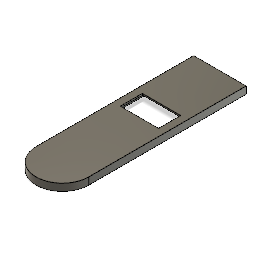
M365_panel_windowed (Autodesk Fusion 360 design; units mm, degrees)
Autodesk Fusion 360 part; units mm, degrees
sketch "Sketch1" plane through (0, 0, 0) normal (0, 1, 0) x (1, 0, 0)
  line L0 (-16.3, 0) -> (16.3, 0)
  line L1 (16.3, 0) -> (16.3, 97.5)
  line L2 (16.3, 97.5) -> (-16.3, 97.5)
  line L3 (-16.3, 97.5) -> (-16.3, 0)
  line L4 (0, 102.6744) -> (0, -20) construction
  arc A0 (-16.3, 0) -> (16.3, 0) centre (0, 0) ccw
  line L5 (-14.35, 97.5) -> (-14.35, 0)
  arc A1 (-14.35, 0) -> (14.35, 0) centre (0, 0) ccw
  line L6 (14.35, 0) -> (14.35, 97.5)
  dimension "d1" = 32.6
  dimension "d2" = 97.5
  dimension "d3" = 1.95
  measures "d3" distance of L3
extrude "Extrude1" add sketch "Sketch1" along normal blind 2
extrude "Extrude2" add sketch "Sketch1" against normal blind 2.5 contours L0 L2 L3 L5 | L0 A0 A1 | L0 L1 L2 L6
sketch "Sketch2" plane through (0, 0, 7.15) normal (0, 1, 0) x (1, 0, 0)
  circle A0 centre (0, 7.15) radius 3.5
  circle A1 centre (0, 7.15) radius 4.1
  circle A2 centre (0, 7.15) radius 4.7
  circle A3 centre (0, 7.15) radius 5.3
  circle A4 centre (0, 7.15) radius 5.9
  circle A5 centre (0, 7.15) radius 6.5
  circle A6 centre (0, 7.15) radius 7.1
  circle A7 centre (0, 7.15) radius 7.7
  circle A8 centre (0, 7.15) radius 8.3
  line L0 (27.1083, -9.4638) -> (28.3083, -9.4638)
  line L1 (28.3083, -9.4638) -> (28.3083, -7.488)
  line L2 (28.3083, -7.488) -> (27.1083, -7.488)
  line L3 (27.1083, -7.488) -> (27.1083, -9.4638)
  circle A9 centre (0, 7.15) radius 8.9
  circle A10 centre (0, 7.15) radius 9.5
  circle A11 centre (0, 7.15) radius 10.1
  circle A12 centre (0, 7.15) radius 10.7
  circle A13 centre (0, 7.15) radius 11.3
  circle A14 centre (0, 7.15) radius 11.9
  circle A15 centre (0, 7.15) radius 12.5
  dimension "d18" = 7
  dimension "d19" = 8.2
  dimension "d20" = 1.2
  dimension "d21" = 9.4
  dimension "d22" = 10.6
  dimension "d23" = 11.8
  dimension "d24" = 13
  dimension "d25" = 14.2
  dimension "d26" = 15.4
  dimension "d27" = 16.6
  dimension "d28" = 17.8
  dimension "d29" = 19
  dimension "d30" = 20.2
  dimension "d31" = 21.4
  dimension "d32" = 22.6
  dimension "d33" = 23.8
  dimension "d34" = 25
  measures "d18" diameter of A0
  measures "d19" diameter of A1
  measures "d21" diameter of A2
  measures "d22" diameter of A3
  measures "d23" diameter of A4
  measures "d24" diameter of A5
  measures "d25" diameter of A6
  measures "d26" diameter of A7
  measures "d27" diameter of A8
  measures "d28" diameter of A9
  measures "d29" diameter of A10
  measures "d30" diameter of A11
  measures "d31" diameter of A12
  measures "d32" diameter of A13
  measures "d33" diameter of A14
  measures "d34" diameter of A15
extrude "Extrude4" cut sketch "Sketch2" along normal blind 1.25 contours A1 | A2 | A3 | A4 | A5 | A6 | A7 | A8 | A9 | A10 | A11 | A12 | A13 | A14 | A15
extrude "Extrude5" add 1 faces at (0.555, 0, 0.9381) along direction (0, -1, 0) blind 1.5
sketch "Sketch3" plane through (0, 0, 0) normal (0, -1, 0) x (1, 0, 0)
  line L0 (14.35, -97.5) -> (14.35, 0)
  arc A0 (14.35, 0) -> (-14.35, 0) centre (0, 0) ccw
  line L1 (-14.35, 0) -> (-14.35, -97.5)
  line L2 (-14.35, -97.5) -> (14.35, -97.5)
  circle A1 centre (0, 0) radius 12.5
  line L3 (13, -62.5) -> (-13, -62.5)
  line L4 (-13, -62.5) -> (-13, -46.5)
  line L5 (-13, -46.5) -> (13, -46.5)
  line L6 (13, -46.5) -> (13, -62.5)
  line L7 (13, -62.5) -> (-13, -46.5) construction
  line L8 (-13, -62.5) -> (13, -46.5) construction
  dimension "d39" = 26
  dimension "d40" = 16
  dimension "d41" = 35
  measures "d41" distance of L2 L3
extrude "Extrude6" cut sketch "Sketch3" against normal blind 1 contours L3 L4 L5 L6
sketch "Sketch4" plane through (0, 1, 0) normal (0, -1, 0) x (1, 0, 0)
  line L0 (13, -46.5) -> (-13, -46.5)
  line L1 (-13, -46.5) -> (-13, -62.5)
  line L2 (-13, -62.5) -> (13, -62.5)
  line L3 (13, -62.5) -> (13, -46.5)
  line L4 (11.8, -61.3) -> (-11.8, -61.3)
  line L5 (-11.8, -61.3) -> (-11.8, -47.7)
  line L6 (-11.8, -47.7) -> (11.8, -47.7)
  line L7 (11.8, -47.7) -> (11.8, -61.3)
  line L8 (11.8, -61.3) -> (-11.8, -47.7) construction
  line L9 (-11.8, -61.3) -> (11.8, -47.7) construction
  dimension "d44" = 23.6
  dimension "d45" = 13.6
extrude "Extrude7" cut sketch "Sketch4" against normal blind 1 contours L4 L5 L6 L7
equation "d1 = 33 mm - 0.4 mm"
equation "d2 = 114 mm - ( 33 / 2 ) * 1 mm"
equation "d19 = d18 + d20"
equation "d21 = d19 + d20"
equation "d22 = d21 + d20"
equation "d23 = d22 + d20"
equation "d24 = d23 + d20"
equation "d25 = d24 + d20"
equation "d26 = d25 + d20"
equation "d27 = d26 + d20"
equation "d28 = d27 + d20"
equation "d29 = d28 + d20"
equation "d30 = d29 + d20"
equation "d31 = d30 + d20"
equation "d32 = d31 + d20"
equation "d33 = d32 + d20"
equation "d34 = d33 + d20"
